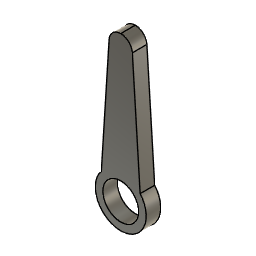
servoaddon (Autodesk Fusion 360 design; units mm, degrees)
Autodesk Fusion 360 part; units mm, degrees
note: some values were not read from the file. Set by a fixed rule: which sketch regions a step uses.
sketch "Sketch1" plane through (0, 31.2, 0) normal (0, 1, 0) x (-1, 0, 0)
  circle A0 centre (0, 5.4143) radius 2.46
  arc A1 (-2.67, 7.6773) -> (2.67, 7.6773) centre (0, 5.4143) ccw
  line L0 (2.67, 7.6773) -> (2.04, 19.8943)
  arc A2 (2.04, 19.8943) -> (-2.04, 19.8943) centre (0, 19.3938) ccw
  line L1 (-2.04, 19.8943) -> (-2.67, 7.6773)
  circle A3 centre (0, 5.4143) radius 2.46
  circle A4 centre (0, 5.4143) radius 3.5
  line L2 (0, 5.4143) -> (0, 25.4143)
  line L3 (0, 25.4143) -> (-1.5, 25.4143)
  line L4 (-1.5, 25.4143) -> (1.5, 25.4143)
  line L5 (1.5, 25.4143) -> (2.67, 7.6773)
  line L6 (-2.67, 7.6773) -> (-1.5, 25.4143)
  dimension "d1" = 20
  dimension "d2" = 1.5
  dimension "d3" = 3
  constraint concentric A0 A3
  constraint concentric A0 A4
  constraint coincident A0.centre A1.centre
  constraint vertical L2
  constraint perpendicular L2 L3
  constraint perpendicular L2 L4
  constraint coincident A1.end L0.start
  constraint coincident A1.start L1.end
  measures "d1" distance of A0.centre L2.end
  measures "d2" distance of L2.end L3.end
  measures "d3" distance of L3.end L4.end
extrude "Extrude1" add sketch "Sketch1" along normal blind 5 contours A1 A4 | A2 A4 L2 L6 | A2 A4 L2 L5 | A2 L2 L3 L4 L6 | A2 L2 L4 L5
extrude "Extrude2" cut 1 faces at (0, 36.2, 16.2426) along direction (0, -1, 0) blind 3
move_body "Move1" bodies 1 to x (1, 0, 0) y (0, 1, 0) z (0, 0, 1) at (16, 0, 0)
fillet "Fillet1" radius 1.6 2 edges at (14.5, 32.2, 25.4143) (17.5, 32.2, 25.4143)
